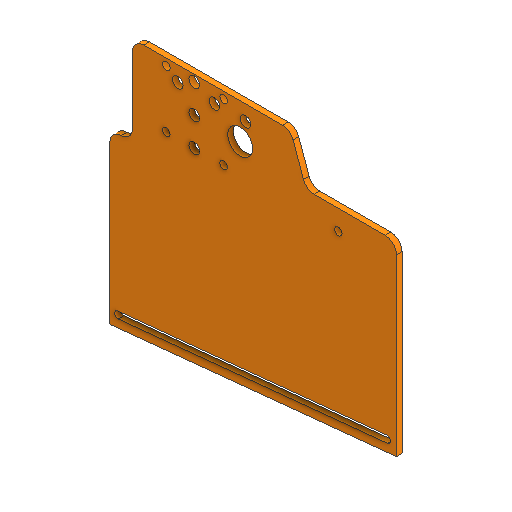
# Autodesk Inventor part: CHAPA FIXAÇÃO DIREITA 1
Saved by Autodesk Inventor 2027.1 (Build 311270010, 270A)
## iProperties
Created: 2026-08-12
Part Number: CHAPA FIXAÇÃO DIREITA 1
Material: Genérico
Document SubType Name: Modeling
Designer: djair.oliveira
Density: 1 g/cm^3
Appearance: Padrão
Author: djair.oliveira
Autodesk Inventor part; units mm, degrees
ref_plane "YZ Plane" through (0, 0, 0) normal (1, 0, 0) x (0, 1, 0)
ref_plane "XZ Plane" through (0, 0, 0) normal (0, 1, 0) x (-1, 0, 0)
ref_plane "XY Plane" through (0, 0, 0) normal (0, 0, 1) x (1, 0, 0)
sketch "Esboço1" plane through (0, 0, 0) normal (0, 0, 1) x (1, 0, 0)
  line L0 (136.913, 75.5114) -> (56.913, 75.5114)
  line L1 (56.913, 75.5114) -> (42.913, 114.5391)
  line L2 (42.913, 114.5391) -> (-117.087, 114.5391)
  line L3 (-117.087, 114.5391) -> (-117.087, -114.7608)
  line L4 (136.913, 75.5114) -> (136.913, -89.3608)
  line L5 (136.913, -89.3608) -> (-117.087, -114.7608)
  line L6 (136.913, 46.0024) -> (136.913, 42.8274)
  line L7 (-116.1736, -114.6695) -> (137.8264, -89.2695)
  circle A0 centre (85.351, 57.8134) radius 3.3782
  circle A1 centre (-42.3105, 57.8134) radius 4.7625
  circle A2 centre (-42.3105, 83.2134) radius 4.7625
  circle A3 centre (-56.9241, 100.9934) radius 4.7625
  circle A4 centre (-24.4105, 100.9934) radius 4.7625
  circle A5 centre (-42.3105, 108.6134) radius 4.7625
  circle A6 centre (-67.049, 57.8134) radius 3.3782
  circle A7 centre (-1.5943, 83.2134) radius 11.1125
  circle A8 centre (-16.249, 57.8134) radius 3.3782
  circle A9 centre (3.0987, 100.9934) radius 4.7625
  circle A10 centre (-16.249, 108.6134) radius 3.3782
  circle A11 centre (-67.049, 108.6134) radius 3.3782
  circle A12 centre (-117.849, 57.8134) radius 6.096
  line L8 (129.1695, -83.1003) -> (-109.6394, -106.9812)
  arc A13 (129.1695, -83.1003) -> (128.5725, -77.1301) centre (128.871, -80.1152) ccw
  line L9 (-110.2364, -101.011) -> (128.5725, -77.1301)
  arc A14 (-110.2364, -101.011) -> (-109.6394, -106.9812) centre (-109.9379, -103.9961) ccw
  line L10 (-97.087, 114.5391) -> (-117.087, 114.5391)
  line L11 (-117.087, 114.5391) -> (-117.087, 35.1191)
  line L12 (-117.087, 35.1191) -> (-97.087, 35.1191)
  line L13 (-97.087, 35.1191) -> (-97.087, 114.5391)
  point P0 (0, 0)
  point P1 (-117.087, 63.8616)
  point P2 (-117.087, 51.7652)
  dimension "d0" = 254
  dimension "d1" = 80
  dimension "d2" = 160
  dimension "d3" = 109.734
  dimension "d6" = 20
  constraints: 28 end point, 15 centre point, 4 point on circle, 3 collinear, 3 parallel, 2 horizontal, 2 perpendicular, 2 point on line, 1 vertical
  measures "d0" distance between parallel lines of L4 L3
  measures "d1" distance of L0.start L0.end
  measures "d2" distance of L1.end L2.end
  measures "d3" angle of L2 L1
  measures "d6" distance between parallel lines of L3 L13
extrude "Extrusão1" add sketch "Esboço1" along normal blind 5 contours L4 L5 L3 L12 L13 L2 L1 L0
fillet "Arredondamento1" radius 10 6 edges at (-97.087, 35.1191, 2.5) (-117.087, 35.1191, 2.5) (-97.087, 114.5391, 2.5) (42.913, 114.5391, 2.5) (56.913, 75.5114, 2.5) (136.913, 75.5114, 2.5)
